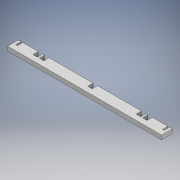
# Autodesk Inventor part: brace
Saved by Autodesk Inventor 2017 (Build 210142000, 142)
## iProperties
Created: 2017-05-14
Part Number: brace
Material: Generic
Document SubType Name: Modeling
Designer: s4461999
Density: 1 g/cm^3
Appearance: Default
Author: s4461999
Autodesk Inventor part; units mm, degrees
ref_plane "YZ Plane" through (0, 0, 0) normal (1, 0, 0) x (0, 1, 0)
ref_plane "XZ Plane" through (0, 0, 0) normal (0, 1, 0) x (-1, 0, 0)
ref_plane "XY Plane" through (0, 0, 0) normal (0, 0, 1) x (1, 0, 0)
sketch "Sketch1" plane through (0, 0, 0) normal (0, 0, 1) x (1, 0, 0)
  line L0 (0, 0) -> (143.2, 0)
  line L1 (143.2, 0) -> (143.2, 20)
  line L2 (143.2, 20) -> (138.2, 20)
  line L3 (138.2, 20) -> (138.2, 10)
  line L4 (138.2, 10) -> (135, 10)
  line L5 (135, 10) -> (135, 20)
  line L6 (135, 20) -> (106.1, 20)
  line L7 (106.1, 20) -> (106.1, 10)
  line L8 (106.1, 10) -> (97.9, 10)
  line L9 (97.9, 10) -> (97.9, 20)
  line L10 (97.9, 20) -> (94.3, 20)
  line L11 (94.3, 20) -> (94.3, 10)
  line L12 (94.3, 10) -> (86.1, 10)
  line L13 (86.1, 10) -> (86.1, 20)
  line L14 (86.1, 20) -> (4.1, 20)
  line L15 (4.1, 20) -> (4.1, 10)
  line L16 (4.1, 10) -> (0, 10)
  line L17 (0, 50) -> (0, 0)
  line L18 (0, 0) -> (-143.2, 0)
  line L19 (-143.2, 0) -> (-143.2, 20)
  line L20 (-143.2, 20) -> (-138.2, 20)
  line L21 (-138.2, 20) -> (-138.2, 10)
  line L22 (-138.2, 10) -> (-135, 10)
  line L23 (-135, 10) -> (-135, 20)
  line L24 (-135, 20) -> (-106.1, 20)
  line L25 (-106.1, 20) -> (-106.1, 10)
  line L26 (-106.1, 10) -> (-97.9, 10)
  line L27 (-97.9, 10) -> (-97.9, 20)
  line L28 (-97.9, 20) -> (-94.3, 20)
  line L29 (-94.3, 20) -> (-94.3, 10)
  line L30 (-94.3, 10) -> (-86.1, 10)
  line L31 (-86.1, 10) -> (-86.1, 20)
  line L32 (-86.1, 20) -> (-4.1, 20)
  line L33 (-4.1, 20) -> (-4.1, 10)
  line L34 (-4.1, 10) -> (0, 10)
  dimension "d4" = 3.2
  dimension "d5" = 20
  dimension "d6" = 10
  dimension "d7" = 0
  dimension "d8" = 82
  dimension "d9" = 0
  dimension "d10" = 135
  dimension "d11" = 20
  dimension "d12" = 5
  dimension "d13" = 8.2
  dimension "d14" = 8.2
  dimension "d15" = 4.1
  dimension "d16" = 50
  constraints: 70 end point, 18 point on line, 16 symmetric about line, 11 perpendicular, 2 coincident, 2 horizontal, 1 vertical
  measures "d4" distance between parallel lines of L3 L5
  measures "d5" distance between parallel lines of L2 L0
  measures "d6" distance of L2.end L3.end
  measures "d7" distance between parallel lines of L12 L16
  measures "d8" distance between parallel lines of L13 L15
  measures "d9" horizontal distance of L0.start L16.end
  measures "d10" distance from line of L5 L0.start
  measures "d11" distance between parallel lines of L13 L7
  measures "d12" distance of L1.end L2.end
  measures "d13" distance between parallel lines of L11 L13
  measures "d14" distance between parallel lines of L7 L9
  measures "d15" distance of L15.end L16.end
  measures "d16" distance of L17.start L17.end
extrude "Extrusion1" add sketch "Sketch1" along normal blind 8
body "Solid1"
